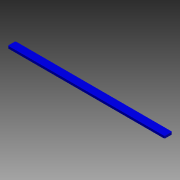
# Autodesk Inventor part: OpenROV 2_3 Dev Bulkhead Brace
Saved by Autodesk Inventor 2012 (Build 160160000, 160)
## iProperties
Created: 2012-05-10
Part Number: OpenROV 2_3 Dev Bulkhead Brace
Material: Default
Document SubType Name: Modeling
Designer: user
Density: 1 g/cm^3
Author: user
Autodesk Inventor part; units mm, degrees
ref_plane "YZ Plane" through (0, 0, 0) normal (1, 0, 0) x (0, 1, 0)
ref_plane "XZ Plane" through (0, 0, 0) normal (0, 1, 0) x (-1, 0, 0)
ref_plane "XY Plane" through (0, 0, 0) normal (0, 0, 1) x (1, 0, 0)
sketch "Sketch1" plane through (0, 0, 0) normal (0, 0, 1) x (1, 0, 0)
  line L0 (1, 0) -> (205, 0)
  line L1 (206, 1) -> (206, 9)
  line L2 (205, 10) -> (1, 10)
  line L3 (0, 9) -> (0, 1)
  arc A0 (205, 0) -> (206, 1) centre (205, 1) ccw
  arc A1 (206, 9) -> (205, 10) centre (205, 9) ccw
  arc A2 (1, 10) -> (0, 9) centre (1, 9) ccw
  arc A3 (0, 1) -> (1, 0) centre (1, 1) ccw
  point P0 (0, 0)
  point P1 (206, 10)
  point P2 (0, 10)
  dimension "d0" = 10
  dimension "d1" = 206
  dimension "d2" = 1
  dimension "d5" = 1
  constraints: 8 end point, 8 point on circle, 8 tangent, 6 point on line, 4 centre point, 2 equal radius, 2 parallel, 1 horizontal, 1 perpendicular
  measures "d0" distance between parallel lines of L0 L2
  measures "d1" distance between parallel lines of L1 L3
  measures "d2" radius of A0
  measures "d5" radius of A1
extrude "Extrusion1" add sketch "Sketch1" along normal blind 3
body "Solid1"
